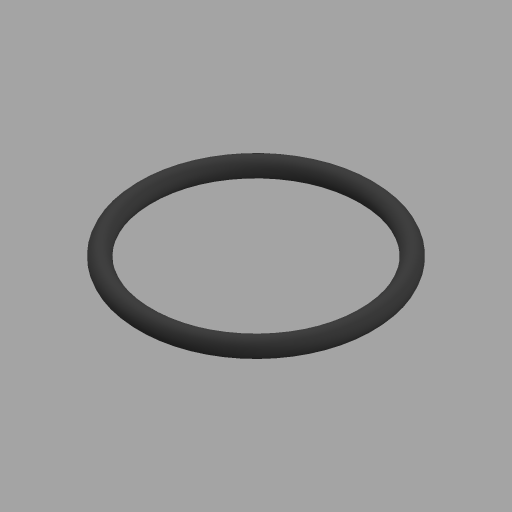
# Autodesk Inventor part: oring
Saved by Autodesk Inventor 2024 (Build 280153020, 153B)
## iProperties
Created: 2023-11-04
Part Number: oring
Material: Rubber
Document SubType Name: Modeling
Designer: schanen
Density: 0.93 g/cm^3
Appearance: Rubber - Black
Mass: 1.77884 g
Surface Area: 19.1273 cm^2
Volume: 1.91273 cm^3
oring_dia: 4.000 mm
oring_id: 45.000 mm
oring_od: 53.000 mm
Author: schanen
Autodesk Inventor part; units mm, degrees
ref_plane "YZ Plane" through (0, 0, 0) normal (1, 0, 0) x (0, 1, 0)
ref_plane "XZ Plane" through (0, 0, 0) normal (0, 1, 0) x (-1, 0, 0)
ref_plane "XY Plane" through (0, 0, 0) normal (0, 0, 1) x (1, 0, 0)
sketch "Sketch1" plane through (0, 0, 0) normal (0, 0, 1) x (1, 0, 0)
  circle A0 centre (-24.5, 0) radius 2
  line L0 (0, -2.8) -> (0, 2.8) projected
  point P0 (0, 0)
  dimension "oring_dia" = 4
  dimension "d3" = 24.5
  constraints: 1 centre point
  measures "oring_dia" diameter of A0
  measures "d3" distance from line of L0 A0.centre
revolve "Revolution1" add sketch "Sketch1" angle 360 about axis through (0, -10, 0) along (0, 1, 0)
equation "\"d3\" = oring_ir + 0.5 * oring_dia"
equation "\"oring_id\" = 2 * oring_ir"
equation "\"oring_od\" = oring_id + 2 * oring_dia"
equation "\"oring_ir\" = 22.5"
body "Solid1"
